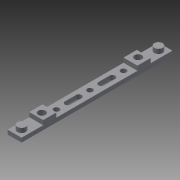
# Autodesk Inventor part: roller_holder_2
Saved by Autodesk Inventor 2015 (Build 190159000, 159)
## iProperties
Created: 2017-12-05
Part Number: roller_holder_2
Material: Generic
Document SubType Name: Modeling
Designer: Anshul
Density: 1 g/cm^3
Appearance: Default
Author: Anshul
Autodesk Inventor part; units mm, degrees
ref_plane "YZ Plane" through (0, 0, 0) normal (1, 0, 0) x (0, 1, 0)
ref_plane "XZ Plane" through (0, 0, 0) normal (0, 1, 0) x (-1, 0, 0)
ref_plane "XY Plane" through (0, 0, 0) normal (0, 0, 1) x (1, 0, 0)
sketch "Sketch1" plane through (0, 0, 0) normal (0, 1, 0) x (-1, 0, 0)
  line L0 (0, 0) -> (0, -100)
  line L1 (10, -100) -> (10, 0)
  circle A0 centre (5, -84.5) radius 2.6
  circle A1 centre (5, -15.5) radius 2.6
  circle A2 centre (5, -1) radius 3
  line L2 (10, 0) -> (10, 4)
  line L3 (10, 4) -> (0, 4)
  line L4 (0, 4) -> (0, 0)
  line L5 (10, -100) -> (10, -104)
  line L6 (10, -104) -> (0, -104)
  line L7 (0, -104) -> (0, -100)
  circle A3 centre (5, -99) radius 3
  circle A4 centre (5, -26) radius 2
  arc A5 (7, -34) -> (3, -34) centre (5, -34) ccw
  arc A6 (3, -42) -> (7, -42) centre (5, -42) ccw
  circle A7 centre (5, -50) radius 2
  arc A8 (7, -58) -> (3, -58) centre (5, -58) ccw
  arc A9 (3, -66) -> (7, -66) centre (5, -66) ccw
  circle A10 centre (5, -74) radius 2
  line L8 (7, -34) -> (7, -42)
  line L9 (3, -34) -> (3, -42)
  line L10 (7, -58) -> (7, -66)
  line L11 (3, -58) -> (3, -66)
  line L12 (5, -21) -> (10, -21)
  line L13 (5, -21) -> (0, -21)
  line L14 (5, -11.5) -> (10, -11.5)
  line L15 (5, -11.5) -> (0, -11.5)
  line L16 (5, -79) -> (10, -79)
  line L17 (5, -79) -> (0, -79)
  line L18 (5, -88.5) -> (10, -88.5)
  line L19 (5, -88.5) -> (0, -88.5)
  dimension "d0" = 100
  dimension "d1" = 10
  dimension "d4" = 5.2
  dimension "d7" = 5.2
  dimension "d9" = 6
  dimension "d10" = 4
  dimension "d11" = 4
  dimension "d13" = 6
  dimension "d20" = 4
  dimension "d21" = 4
  dimension "d22" = 4
  dimension "d23" = 4
  dimension "d24" = 4
  dimension "d25" = 4
  dimension "d26" = 4
  dimension "d27" = 5.5
  dimension "d28" = 4
  dimension "d29" = 5.5
  dimension "d30" = 4
  constraints: 40 end point, 18 point on line, 11 centre point, 8 point on circle, 7 perpendicular, 2 tangent, 2 vertical, 1 parallel
  measures "d0" distance of L0.start L0.end
  measures "d1" distance of L0.end L1.start
  measures "d4" diameter of A0
  measures "d7" diameter of A1
  measures "d9" diameter of A2
  measures "d10" distance of L1.end L2.end
  measures "d11" distance of L1.start L5.end
  measures "d13" diameter of A3
  measures "d20" diameter of A4
  measures "d21" diameter of A5
  measures "d22" diameter of A6
  measures "d23" diameter of A7
  measures "d24" diameter of A8
  measures "d25" diameter of A9
  measures "d26" diameter of A10
  measures "d27" distance of A1.centre L12.start
  measures "d28" distance of A1.centre L14.start
  measures "d29" distance of A0.centre L16.start
  measures "d30" distance of A0.centre L18.start
extrude "Extrusion1" add sketch "Sketch1" along normal blind 3 contours L4 L3 L2 L1 L14 L15 L0 | L13 L12 L1 L16 L17 L0 | L19 L18 L1 L5 L6 L7 L0
extrude "Extrusion2" add sketch "Sketch1" along normal blind 6.2 contours L15 L14 L1 L12 L13 L0 | L17 L16 L1 L18 L19 L0 | A2 | A3
body "Solid1"
